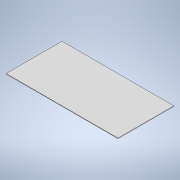
# Autodesk Inventor part: wire_holder_lasercutting800
Saved by Autodesk Inventor 2021 (Build 250183000, 183)
## iProperties
Created: 2021-02-03
Part Number: wire_holder_lasercutting800
Material: Generic
Document SubType Name: Modeling
Designer: User
Density: 1 g/cm^3
Appearance: Default
Author: User
Autodesk Inventor part; units mm, degrees
ref_plane "YZ Plane" through (0, 0, 0) normal (1, 0, 0) x (0, 1, 0)
ref_plane "XZ Plane" through (0, 0, 0) normal (0, 1, 0) x (-1, 0, 0)
ref_plane "XY Plane" through (0, 0, 0) normal (0, 0, 1) x (1, 0, 0)
sketch "Sketch1" plane through (0, 0, 0) normal (0, 1, 0) x (-1, 0, 0)
  line L0 (-17.9221, -16.5) -> (-498.4221, -16.5)
  line L1 (-518.4221, 3.5) -> (-518.4221, 130)
  line L2 (-498.4221, 150) -> (251.5779, 150)
  line L3 (271.5779, 130) -> (271.5779, 30)
  line L4 (-18.4221, -12) -> (-498.4221, -12)
  line L5 (-513.9221, 3.5) -> (-513.9221, 130)
  line L6 (-498.4221, 145.5) -> (251.5779, 145.5)
  line L7 (267.0779, 130) -> (267.0779, 30)
  line L8 (251.5779, 14.5) -> (-488.9221, 14.5)
  line L9 (-504.4221, 30) -> (-504.4221, 120.5)
  line L10 (251.5779, 10) -> (-488.9221, 10)
  line L11 (-508.9221, 30) -> (-508.9221, 120.5)
  line L12 (-488.9221, 136) -> (242.0779, 136)
  line L13 (-488.9221, 140.5) -> (242.0779, 140.5)
  line L14 (257.5779, 120.5) -> (257.5779, 56.5)
  line L15 (242.0779, 41) -> (-479.4221, 41)
  line L16 (262.0779, 120.5) -> (262.0779, 56.5)
  line L17 (242.0779, 36.5) -> (-479.4221, 36.5)
  line L18 (-494.9221, 56.5) -> (-494.9221, 111)
  line L19 (-479.4221, 126.5) -> (232.5779, 126.5)
  line L20 (248.0779, 111) -> (248.0779, 83)
  line L21 (232.5779, 67.5) -> (-488.9221, 67.5)
  line L22 (-499.4221, 56.5) -> (-499.4221, 111)
  line L23 (-479.4221, 131) -> (232.5779, 131)
  line L24 (252.5779, 111) -> (252.5779, 83)
  line L25 (232.5779, 63) -> (-488.9221, 63)
  line L26 (-122.9221, 150) -> (-122.9221, -150) construction
  line L27 (-18.9221, -12) -> (251.5779, -12)
  line L28 (271.5779, -32) -> (271.5779, -129.5)
  line L29 (251.5779, -149.5) -> (-498.4221, -149.5)
  line L30 (-518.4221, -129.5) -> (-518.4221, -58.5)
  line L31 (-18.9221, -16.5) -> (251.5779, -16.5)
  line L32 (267.0779, -32) -> (267.0779, -129.5)
  line L33 (251.5779, -145) -> (-498.4221, -145)
  line L34 (-498.4221, -38.5) -> (242.0779, -38.5)
  line L35 (262.0779, -58.5) -> (262.0779, -120)
  line L36 (242.0779, -140) -> (-488.9221, -140)
  line L37 (-513.9221, -129.5) -> (-513.9221, -58.5)
  line L38 (-498.4221, -43) -> (242.0779, -43)
  line L39 (257.5779, -58.5) -> (257.5779, -120)
  line L40 (242.0779, -135.5) -> (-488.9221, -135.5)
  line L41 (-504.4221, -120) -> (-504.4221, -85)
  line L42 (-508.9221, -120) -> (-508.9221, -85)
  line L43 (-488.9221, -65) -> (232.5779, -65)
  line L44 (252.5779, -85) -> (252.5779, -110.5)
  line L45 (-488.9221, -69.5) -> (232.5779, -69.5)
  line L46 (248.0779, -85) -> (248.0779, -110.5)
  line L47 (232.5779, -126) -> (-488.9221, -126)
  line L48 (232.5779, -130.5) -> (-488.9221, -130.5)
  line L49 (276.5779, 200.5) -> (276.5779, -199.5)
  line L50 (276.5779, -199.5) -> (-523.4221, -199.5)
  line L51 (-523.4221, -199.5) -> (-523.4221, 200)
  line L52 (-523.4221, 200) -> (276.5779, 200)
  line L53 (276.5779, 200) -> (276.5779, -199.5)
  arc A0 (251.5779, -149.5) -> (271.5779, -129.5) centre (251.5779, -129.5) ccw
  arc A1 (251.5779, -145) -> (267.0779, -129.5) centre (251.5779, -129.5) ccw
  arc A2 (242.0779, -135.5) -> (257.5779, -120) centre (242.0779, -120) ccw
  arc A3 (242.0779, -140) -> (262.0779, -120) centre (242.0779, -120) ccw
  arc A4 (232.5779, -130.5) -> (252.5779, -110.5) centre (232.5779, -110.5) ccw
  arc A5 (232.5779, -126) -> (248.0779, -110.5) centre (232.5779, -110.5) ccw
  arc A6 (248.0779, -85) -> (232.5779, -69.5) centre (232.5779, -85) ccw
  arc A7 (252.5779, -85) -> (232.5779, -65) centre (232.5779, -85) ccw
  line L54 (266.0656, -58.5) -> (242.0779, -58.5) construction
  line L55 (242.0779, -58.5) -> (242.0779, -27) construction
  arc A8 (257.5779, -58.5) -> (242.0779, -43) centre (242.0779, -58.5) ccw
  arc A9 (262.0779, -58.5) -> (242.0779, -38.5) centre (242.0779, -58.5) ccw
  line L56 (251.5779, -3.7302) -> (251.5779, -32) construction
  line L57 (251.5779, -32) -> (272.6377, -32) construction
  arc A10 (267.0779, -32) -> (251.5779, -16.5) centre (251.5779, -32) ccw
  arc A11 (271.5779, -32) -> (251.5779, -12) centre (251.5779, -32) ccw
  arc A12 (-518.4221, -129.5) -> (-498.4221, -149.5) centre (-498.4221, -129.5) ccw
  arc A13 (-513.9221, -129.5) -> (-498.4221, -145) centre (-498.4221, -129.5) ccw
  arc A14 (-508.9221, -120) -> (-488.9221, -140) centre (-488.9221, -120) ccw
  line L58 (-488.9221, -130.5) -> (-488.9221, -126)
  arc A15 (-504.4221, -120) -> (-488.9221, -135.5) centre (-488.9221, -120) ccw
  arc A16 (-488.9221, -65) -> (-508.9221, -85) centre (-488.9221, -85) ccw
  arc A17 (-488.9221, -69.5) -> (-504.4221, -85) centre (-488.9221, -85) ccw
  arc A18 (-498.4221, -43) -> (-513.9221, -58.5) centre (-498.4221, -58.5) ccw
  arc A19 (-498.4221, -38.5) -> (-518.4221, -58.5) centre (-498.4221, -58.5) ccw
  line L59 (-488.9221, 63) -> (-488.9221, 67.5)
  arc A20 (-518.4221, 3.5) -> (-498.4221, -16.5) centre (-498.4221, 3.5) ccw
  arc A21 (-513.9221, 3.5) -> (-498.4221, -12) centre (-498.4221, 3.5) ccw
  arc A22 (-508.9221, 30) -> (-488.9221, 10) centre (-488.9221, 30) ccw
  arc A23 (-504.4221, 30) -> (-488.9221, 14.5) centre (-488.9221, 30) ccw
  arc A24 (-499.4221, 56.5) -> (-479.4221, 36.5) centre (-479.4221, 56.5) ccw
  arc A25 (-494.9221, 56.5) -> (-479.4221, 41) centre (-479.4221, 56.5) ccw
  arc A26 (-479.4221, 126.5) -> (-494.9221, 111) centre (-479.4221, 111) ccw
  arc A27 (-479.4221, 131) -> (-499.4221, 111) centre (-479.4221, 111) ccw
  arc A28 (-488.9221, 136) -> (-504.4221, 120.5) centre (-488.9221, 120.5) ccw
  arc A29 (-488.9221, 140.5) -> (-508.9221, 120.5) centre (-488.9221, 120.5) ccw
  arc A30 (-498.4221, 145.5) -> (-513.9221, 130) centre (-498.4221, 130) ccw
  arc A31 (-498.4221, 150) -> (-518.4221, 130) centre (-498.4221, 130) ccw
  arc A32 (251.5779, 10) -> (271.5779, 30) centre (251.5779, 30) ccw
  arc A33 (251.5779, 14.5) -> (267.0779, 30) centre (251.5779, 30) ccw
  arc A34 (242.0779, 41) -> (257.5779, 56.5) centre (242.0779, 56.5) ccw
  arc A35 (242.0779, 36.5) -> (262.0779, 56.5) centre (242.0779, 56.5) ccw
  arc A36 (232.5779, 63) -> (252.5779, 83) centre (232.5779, 83) ccw
  arc A37 (232.5779, 67.5) -> (248.0779, 83) centre (232.5779, 83) ccw
  arc A38 (248.0779, 111) -> (232.5779, 126.5) centre (232.5779, 111) ccw
  arc A39 (252.5779, 111) -> (232.5779, 131) centre (232.5779, 111) ccw
  arc A40 (257.5779, 120.5) -> (242.0779, 136) centre (242.0779, 120.5) ccw
  arc A41 (262.0779, 120.5) -> (242.0779, 140.5) centre (242.0779, 120.5) ccw
  arc A42 (267.0779, 130) -> (251.5779, 145.5) centre (251.5779, 130) ccw
  arc A43 (271.5779, 130) -> (251.5779, 150) centre (251.5779, 130) ccw
  circle A44 centre (-493.4221, -169.5) radius 3.25
  circle A45 centre (246.5779, 170) radius 3.25
  point P0 (-228.4221, 0)
  point P1 (276.5779, 200)
  point P2 (257.5779, -126)
  dimension "d2" = 4.5
  dimension "d3" = 4.5
  dimension "d4" = 4.5
  dimension "d5" = 5
  dimension "d6" = 5
  dimension "d7" = 4.5
  dimension "d8" = 4.5
  dimension "d9" = 4.5
  dimension "d10" = 5
  dimension "d11" = 790
  dimension "d12" = 22
  dimension "d13" = 4.5
  dimension "d14" = 4.5
  dimension "d15" = 22
  dimension "d16" = 5
  dimension "d17" = 5
  dimension "d18" = 4.5
  dimension "d19" = 5
  dimension "d20" = 22
  dimension "d21" = 4.5
  dimension "d22" = 4.5
  dimension "d23" = 4.5
  dimension "d30" = 4.5
  dimension "d31" = 4.5
  dimension "d32" = 4.5
  dimension "d34" = 500
  dimension "d35" = 4.5
  dimension "d36" = 4.5
  dimension "d38" = 4.5
  dimension "d39" = 22
  dimension "d40" = 4.5
  dimension "d41" = 5
  dimension "d42" = 4.5
  dimension "d43" = 4.5
  dimension "d44" = 4.5
  dimension "d46" = 22
  dimension "d47" = 5
  dimension "d48" = 4.5
  dimension "d49" = 5
  dimension "d63" = 400
  dimension "d64" = 50
  dimension "d65" = 5
  dimension "d68" = 5
  dimension "d80" = 4.5
  dimension "d81" = 0
  dimension "d103" = 5
  dimension "d126" = 30
  dimension "d127" = 6.5
  dimension "d128" = 30
  dimension "d129" = 6.5
  dimension "d130" = 30
  dimension "d131" = 30
  constraints: 120 end point, 88 point on circle, 46 centre point, 32 perpendicular, 23 coincident, 11 point on line, 10 horizontal, 8 parallel, 6 vertical
  measures "d2" distance between parallel lines of L1 L5
  measures "d3" distance between parallel lines of L2 L6
  measures "d4" distance between parallel lines of L7 L3
  measures "d5" distance between parallel lines of L13 L6
  measures "d6" distance between parallel lines of L5 L11
  measures "d7" distance between parallel lines of L10 L8
  measures "d8" distance between parallel lines of L14 L16
  measures "d9" distance between parallel lines of L13 L12
  measures "d10" distance between parallel lines of L16 L7
  measures "d11" distance between parallel lines of L1 L3
  measures "d12" distance between parallel lines of L4 L10
  measures "d13" distance between parallel lines of L11 L9
  measures "d14" distance between parallel lines of L17 L15
  measures "d15" distance between parallel lines of L8 L17
  measures "d16" distance between parallel lines of L12 L23
  measures "d17" distance between parallel lines of L9 L22
  measures "d18" distance between parallel lines of L23 L19
  measures "d19" distance between parallel lines of L24 L14
  measures "d20" distance between parallel lines of L15 L25
  measures "d21" distance between parallel lines of L24 L20
  measures "d22" distance between parallel lines of L25 L21
  measures "d23" distance between parallel lines of L22 L18
  measures "d30" distance between parallel lines of L31 L27
  measures "d31" distance between parallel lines of L32 L28
  measures "d32" distance between parallel lines of L29 L33
  measures "d34" distance from line of point (-228.422, 0) L28
  measures "d35" distance between parallel lines of L30 L37
  measures "d36" distance between parallel lines of L39 L35
  measures "d38" distance between parallel lines of L34 L38
  measures "d39" distance between parallel lines of L34 L31
  measures "d40" distance between parallel lines of L36 L40
  measures "d41" distance between parallel lines of L33 L36
  measures "d42" distance between parallel lines of L42 L41
  measures "d43" distance between parallel lines of L43 L45
  measures "d44" distance between parallel lines of L46 L44
  measures "d46" distance between parallel lines of L43 L38
  measures "d47" distance between parallel lines of L37 L42
  measures "d48" distance between parallel lines of L48 L47
  measures "d49" distance between parallel lines of L40 L48
  measures "d63" distance of L49.start L49.end
  measures "d64" distance between parallel lines of L50 L29
  measures "d65" distance between parallel lines of L49 L28
  measures "d68" distance between parallel lines of L51 L30
  measures "d80" distance between parallel lines of L4 L0
  measures "d81" distance between parallel lines of L0 L31
  measures "d103" distance between parallel lines of L51 L1
  measures "d126" distance from line of L50 A44.centre
  measures "d127" diameter of A44
  measures "d128" distance from line of L51 A44.centre
  measures "d129" diameter of A45
  measures "d130" distance from line of L53 A45.centre
  measures "d131" distance from line of L52 A45.centre
extrude "Extrusion1" add sketch "Sketch1" along normal blind 4.5 contours L0 A20 L1 A31 L2 A43 L3 A32 L10 A22 L11 A29 L13 A41 L16 A35 L17 A24 L22 A27 L23 A39 L24 A36 L25 L59 L21 A37 L20 A38 L19 A26 L18 A25 L15 A34 L14 A40 L12 A28 L9 A23 L8 A33 L7 A42 L6 A30 L5 A21 L4 L27 A11 L28 A0 L29 A12 L30 A19 L34 A9 L35 A3 L36 A14 L42 A16 L43 A7 L44 A4 L48 L58 L47 A5 L46 A6 L45 A17 L41 A15 L40 A2 L39 A8 L38 A18 L37 A13 L33 A1 L32 A10 L31 | L49 L50 L51 L52 | A44 | A45
equation "\"d6\" = d26"
equation "\"d10\" = d26"
equation "\"d15\" = d28"
equation "\"d16\" = d26"
equation "\"d19\" = d25"
equation "\"d20\" = d28"
equation "\"d34\" = 0.5 * d52"
equation "\"d41\" = d53"
equation "\"d46\" = d54"
equation "\"d47\" = d53"
equation "\"d49\" = d53"
equation "\"d25\" = 5"
equation "\"d26\" = 5"
equation "\"d28\" = -1.2 * d25 + 0.2 * d29"
equation "\"d51\" = 5"
equation "\"d53\" = 5"
equation "\"d54\" = -1.2 * d51 + 0.2 * d55"
equation "\"d29\" = 140"
equation "\"d55\" = 140"
equation "\"d52\" = 1000"
body "Solid1"
